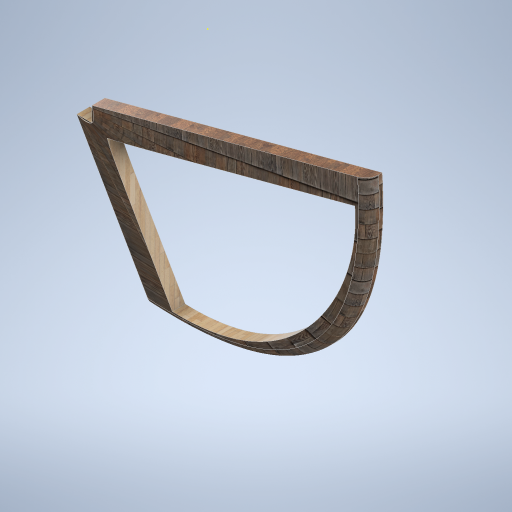
# Autodesk Inventor part: side_curve_corner_frame
Saved by Autodesk Inventor 2024.2 (Build 282272000, 272)
## iProperties
Created: 2024-05-24
Part Number: side_curve_corner_frame
Material: Wood (Maple)
Document SubType Name: Modeling
Designer: LOSTER_1
Density: 0.67 g/cm^3
Appearance: Natural Maple - Glossy Dark Tint
Author: LOSTER_1
Autodesk Inventor part; units mm, degrees
ref_plane "YZ Plane" through (0, 0, 0) normal (1, 0, 0) x (0, 1, 0)
ref_plane "XZ Plane" through (0, 0, 0) normal (0, 1, 0) x (-1, 0, 0)
sketch "Sketch1" plane through (0, 0, 0) normal (1, 0, 0) x (0, 1, 0)
  line L0 (80.2064, 1512.1884) -> (80.2064, 1362.1884)
  line L1 (-94.7936, 1362.1884) -> (-94.7936, 1512.1884)
  line L2 (-94.7936, 1512.1884) -> (80.2064, 1512.1884)
  line L3 (80.2064, 1362.1884) -> (-94.7936, 1362.1884)
  point P0 (0, 0)
  dimension "d0" = 175
  dimension "d1" = 150
  constraints: 8 end point, 1 horizontal, 1 perpendicular
  measures "d0" distance of L1.end L0.start
  measures "d1" distance of L0.start L0.end
ref_plane "Work Plane2" through (2349, 80.2064, 1512.1884) normal (-1, 0, 0) x (0, 0, -1)
ref_plane "Work Plane1" through (0, 80.2064, 1512.1884) normal (-1, 0, 0) x (0, 0, -1)
sketch "Sketch2" plane through (2349, 80.2064, 1512.1884) normal (-1, 0, 0) x (0, 0, -1)
  line L0 (0, 0) -> (150, 0) projected
  point P0 (1512.1884, 80.2064)
ref_plane "Work Plane3" through (2349, 80.2064, 1512.1884) normal (0, 1, 0) x (0, 0, -1)
sketch "Sketch3" plane through (2349, 80.2064, 1512.1884) normal (0, 1, 0) x (0, 0, -1)
  line L0 (0, 0) -> (150, 0) projected
  line L1 (0, 2349) -> (854.9661, 0)
  line L2 (0, 2349) -> (2499.7536, 2349) construction
  line L3 (150, 2349) -> (0, 2349)
  line L4 (150, 2349) -> (1004.9661, 0)
  line L5 (150, 2349) -> (2649.7536, 2349) construction
  line L6 (1004.9661, 0) -> (854.9661, 0)
  point P0 (1512.1884, 2349)
  dimension "d3" = 70
  dimension "d4" = 70
  constraints: 12 end point, 2 equal length, 2 horizontal, 1 collinear, 1 parallel
  measures "d3" angle of L1 L2
  measures "d4" angle of L4 L5
extrude "Extrusion1" add sketch "Sketch3" against normal blind 175
sketch "Sketch4" plane through (2349, -94.7936, 1512.1884) normal (0, -1, 0) x (1, 0, 0)
  line L0 (0, -854.9661) -> (-2349, 0) construction
  line L1 (-2349, 0) -> (-2524, 0) construction
  line L2 (-2524, 0) -> (-2524, -150) construction
  line L3 (-2524, -150) -> (-2349, -150) construction
  line L4 (-2349, -150) -> (-2349, 0) construction
  point P0 (-2349, -1512.1884)
  dimension "d7" = 175
  dimension "d8" = 150
  constraints: 8 end point, 2 parallel, 1 horizontal, 1 perpendicular
  measures "d7" distance of L3.end L2.end
  measures "d8" distance of L2.end L1.end
ref_plane "Work Plane4" through (2349, -2443.7936, 1512.1884) normal (0, -1, 0) x (1, 0, 0)
sketch "Sketch5" plane through (2349, -2443.7936, 1512.1884) normal (0, -1, 0) x (1, 0, 0)
  line L0 (-2524, 0) -> (-2524, -150) construction
  point P0 (-2349, -1512.1884)
ref_plane "Work Plane5" through (-175, -94.7936, 1512.1884) normal (-1, 0, 0) x (0, 0, -1)
sketch "Sketch6" plane through (-175, -94.7936, 1512.1884) normal (-1, 0, 0) x (0, 0, -1)
  line L0 (0, 2349) -> (150, 2349) construction
  line L1 (0, 0) -> (854.9661, 2349) construction
  line L2 (150, 0) -> (1004.9661, 2349) construction
  line L3 (150, 0) -> (2649.7536, 0) construction
  line L4 (1004.9661, 2349) -> (854.9661, 2349) construction
  line L5 (0, 0) -> (150, 0)
  line L6 (0, 0) -> (854.9661, 2349)
  line L7 (1004.9661, 2349) -> (854.9661, 2349)
  line L8 (1004.9661, 2349) -> (150, 0)
  point P0 (1512.1884, -94.7936)
  dimension "d11" = 70
  constraints: 16 end point, 4 horizontal, 1 collinear, 1 equal length
  measures "d11" angle of L3 L2
extrude "Extrusion2" add sketch "Sketch6" against normal blind 175
ref_plane "Work Plane6" through (0, 0, 0) normal (0, 0, 1) x (1, 0, 0)
sketch "Sketch7" plane through (0, 0, 0) normal (0, 0, 1) x (1, 0, 0)
  line L0 (2349, -94.7936) -> (0, -94.7936) projected
  line L1 (0, -94.7936) -> (0, -2443.7936) projected
  arc A0 (0, -2443.7936) -> (2349, -94.7936) centre (386.7502, -481.5438) ccw
  line L2 (0, -94.7936) -> (1800.9638, -1895.7574)
  point P0 (0, 0)
  dimension "d15" = 2000
  constraints: 3 point on circle, 2 end point, 1 centre point
  measures "d15" radius of A0
ref_plane "Work Plane7" through (0, -94.7936, 0) normal (-0.7071068, -0.7071068, 0) x (0.7071068, -0.7071068, 0)
ref_plane "Work Plane8" through (-175, -2443.7936, 507.2224) normal (0, 0, -1) x (1, 0, 0)
sketch "Sketch9" plane through (-175, -2443.7936, 507.2224) normal (0, 0, -1) x (1, 0, 0)
  line L0 (175, -2349) -> (175, 0) projected
  arc A0 (2524, -2349) -> (175, 0) centre (561.7502, -1962.2498) ccw projected
  line L1 (2524, -2349) -> (175, -2349) projected
  point P0 (175, -2443.7936)
sketch "Sketch8" plane through (0, -94.7936, 0) normal (-0.7071068, -0.7071068, 0) x (0.7071068, -0.7071068, 0)
  line L0 (0, 1512.1884) -> (0, 1362.1884) projected
  line L1 (0, 1512.1884) -> (0, 1362.1884)
  line L2 (2546.9474, 507.2224) -> (2546.9474, 657.2224)
  line L3 (0, 1362.1884) -> (2546.9474, 507.2224)
  line L4 (0, 1512.1884) -> (2546.9474, 657.2224)
  point P0 (-67.0292, 0)
  point P1 (1660.9938, 507.2224)
  dimension "d17" = 150
  constraints: 8 end point, 2 vertical
  measures "d17" distance of L2.start L2.end
sketch "Sketch10" plane through (0, -94.7936, 1512.1884) normal (1, 0, 0) x (0, 0, -1)
  line L0 (0, 0) -> (854.9661, -2349) projected
  line L1 (854.9661, -2349) -> (1004.9661, -2349) projected
  line L2 (1004.9661, -2349) -> (150, 0) projected
  line L3 (0, 0) -> (150, 0) projected
  point P0 (1512.1884, 94.7936)
sketch "Sketch11" plane through (2349, -94.7936, 1512.1884) normal (0, -1, 0) x (1, 0, 0)
  line L0 (0, -854.9661) -> (-2349, 0) projected
  line L1 (-2349, 0) -> (-2349, -150) projected
  line L2 (-2349, -150) -> (0, -1004.9661) projected
  line L3 (0, -1004.9661) -> (0, -854.9661) projected
  point P0 (-2349, -1512.1884)
loft "Loft1" add profiles "Sketch8" section 1 edges at (-175, -1269.2936, 1084.7054) (-175, -94.7936, 1437.1884) (-175, -1269.2936, 934.7054) (-175, -2443.7936, 582.2224) section 3 edges at (1174.5, 80.2064, 1084.7054) (2349, 80.2064, 582.2224) (1174.5, 80.2064, 934.7054) (0, 80.2064, 1437.1884)
sketch "Sketch12" plane through (-175, -2443.7936, 507.2224) normal (0, 0, -1) x (1, 0, 0)
  line L0 (175, 0) -> (0, 0) projected
  line L1 (175, -2349) -> (175, 0) projected
  line L2 (2524, -2349) -> (175, -2349) projected
  line L3 (2524, -2524) -> (2524, -2349) projected
  line L4 (175, -2349) -> (295, -2349)
  line L5 (295, -2349) -> (295, -2229)
  line L6 (295, -2229) -> (175, -2229)
  line L7 (175, -2229) -> (175, -2349)
  line L8 (2524, -2349) -> (2404, -2349)
  line L9 (2404, -2349) -> (2404, -2229)
  line L10 (2404, -2229) -> (2524, -2229)
  line L11 (2524, -2229) -> (2524, -2349)
  line L12 (175, 0) -> (295, 0)
  line L13 (295, 0) -> (295, -120)
  line L14 (295, -120) -> (175, -120)
  line L15 (175, -120) -> (175, 0)
  arc A0 (2404, -2229) -> (295, -120) centre (407.1467, -2116.8533) ccw
  line L16 (295, -2229) -> (2404, -2229)
  line L17 (295, -2229) -> (295, -120)
  point P0 (175, -2443.7936)
  dimension "d24" = 120
  dimension "d25" = 120
  dimension "d26" = 120
  dimension "d27" = 120
  dimension "d28" = 120
  dimension "d29" = 120
  dimension "d30" = 2000
  constraints: 28 end point, 6 parallel, 3 horizontal, 3 perpendicular, 2 point on circle, 1 centre point, 1 other
  measures "d24" distance of L6.end L5.end
  measures "d25" distance of L5.end L4.end
  measures "d26" distance of L9.end L10.end
  measures "d27" distance of L8.end L9.end
  measures "d28" distance of L13.end L14.end
  measures "d29" distance of L12.end L13.end
  measures "d30" radius of A0
extrude "Extrusion3" cut sketch "Sketch12" against normal through all contours L17 A0 L16
fillet "Fillet1" radius 150 1 edges at (1800.9638, -1895.7574, 657.2224)
sketch "Sketch14" plane through (-175, -94.7936, 1512.1884) normal (-1, 0, 0) x (0, 0, 1)
  point P0 (-1512.1884, 94.7936)
body "Solid1"
